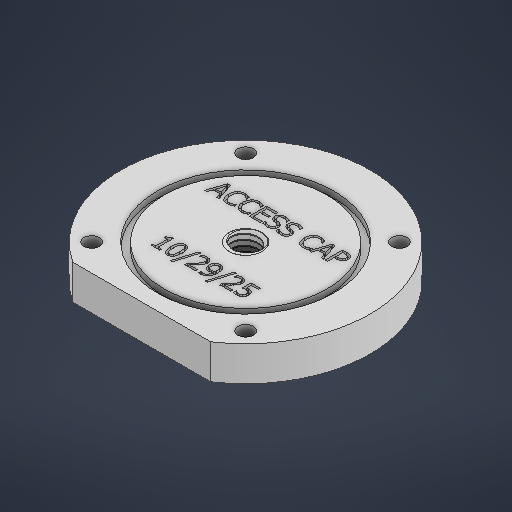
# Autodesk Inventor part: Access Cap
Saved by Autodesk Inventor 2026.2 (Build 302298000, 298)
## iProperties
Created: 2025-10-23
Part Number: Access Cap
Material: Generic
Document SubType Name: Modeling
Designer: mumin
Density: 1 g/cm^3
Appearance: Default
Author: mumin
Autodesk Inventor part; units mm, degrees
ref_plane "YZ Plane" through (0, 0, 0) normal (1, 0, 0) x (0, 1, 0)
ref_plane "XZ Plane" through (0, 0, 0) normal (0, 1, 0) x (-1, 0, 0)
ref_plane "XY Plane" through (0, 0, 0) normal (0, 0, 1) x (1, 0, 0)
sketch "Sketch1" plane through (0, 0, 0) normal (0, 1, 0) x (-1, 0, 0)
  circle A0 centre (0, 0) radius 36
  line L0 (19.8997, 30) -> (-19.8997, 30)
  dimension "d0" = 72
  dimension "d1" = 30
  constraints: 2 end point, 2 point on circle, 1 centre point, 1 coincident, 1 horizontal
  measures "d0" diameter of A0
  measures "d1" distance from line of point (0, 0) L0
extrude "Base" add sketch "Sketch1" along normal blind 10 contours A0 L0 picked at (-0.4083, 8.0069)
sketch "Sketch2" plane through (0, 0, 0) normal (0, -1, 0) x (1, 0, 0)
  circle A0 centre (0, 0) radius 31.4
  line L0 (22.2032, 22.2032) -> (0, 0)
  line L1 (-50.4, 0) -> (50.4, 0) projected
  dimension "d11" = 62.8
  dimension "d12" = 45
  constraints: 2 end point, 1 coincident, 3 other
  measures "d12" angle of L1 L0
hole "Mounting Holes" at (22.2032, 0, 22.2032) direction (0, 1, 0) diameter 4.5 end through all counterbore diameter 8 counterbore depth 4
pattern_circular "Circular Pattern1" count 4 over 360 about axis through (0, 0, 0) along (0, 1, 0) of "Mounting Holes"
sketch "Sketch3" plane through (0, 0, 0) normal (0, 0, 1) x (1, 0, 0)
  line L0 (36, 10) -> (-36, 10) projected
  line L1 (-25.5, 10) -> (-23.5, 10)
  line L2 (-23.5, 10) -> (-23.5, 8.2)
  line L3 (-23.5, 8.2) -> (-25.5, 8.2)
  line L4 (-25.5, 8.2) -> (-25.5, 10)
  line L5 (0, -2) -> (0, 12) projected
  point P0 (0, 0)
  point P1 (19.8997, 10)
  point P2 (-19.8997, 10)
  point P3 (0, 10)
  dimension "d16" = 2
  dimension "d17" = 1.8
  dimension "d18" = 23.5
  constraints: 8 end point, 2 parallel, 1 horizontal, 1 midpoint, 1 perpendicular, 1 point on line
  measures "d16" distance of L2.end L3.end
  measures "d17" distance of L1.end L2.end
  measures "d18" distance from line of point (0, 10) L2
revolve "Seal Groove" cut sketch "Sketch3" angle 360 about axis through (0, -10, 0) along (0, 1, 0)
sketch "Sketch4" plane through (0, 0, 0) normal (0, -1, 0) x (1, 0, 0)
  point P0 (0, 0)
  point P1 (0, 0)
  constraints: 1 coincident
hole "Wire Passthrough" at (0, 0, 0) direction (0, 1, 0) diameter 9.5 end through all
thread "Thread3" size "M10x1.5" class "6H" standard "ANSI Metric M Profile" length 10
sketch "Sketch14" plane through (0, 10, 0) normal (1, 0, 0) x (0, 0, 1)
  line L0 (4.75, 0) -> (4.75, 10)
  line L1 (4.75, 10) -> (3.6378, 10)
  line L2 (3.6378, 10) -> (3.6378, 0)
  line L3 (3.6378, 0) -> (4.75, 0)
  line L4 (0, -3.9629) -> (0, 12.3271) projected
  constraints: 8 end point
revolve "Revolution5" add sketch "Sketch14" angle 360 about axis through (0, 10, 0) along (0, -1, 0) separate body
sketch "Sketch13" plane through (0, 10, 4.75) normal (-1, 0, 0) x (0, -1, 0)
  line L0 (-0.8751, -0.076) -> (-0.7501, -0.076) construction
  line L1 (0.1249, -1.0365) -> (-0.0001, -1.2766) construction
  line L2 (-1.5001, -1.2766) -> (-1.6251, -1.0365) construction
  line L3 (-0.6251, -0.076) -> (-0.7501, 0.1641) construction
  line L4 (-0.7501, 0.1641) -> (-0.8751, -0.076) construction
  line L5 (-1.5001, -1.2766) -> (-1.3751, -1.0365) construction
  line L6 (-0.6251, -0.076) -> (-0.1251, -1.0365)
  line L7 (-1.6251, -1.0365) -> (-1.3751, -1.0365) construction
  arc A0 (-1.6251, -1.0365) -> (-1.5001, -1.1124) centre (-1.5001, -0.9714) ccw construction
  line L8 (0.1249, -1.0365) -> (-0.1251, -1.0365) construction
  line L9 (-1.5001, -1.2766) -> (-1.5001, -1.0365) construction
  line L10 (-0.0001, -1.2766) -> (-0.0001, -1.0365) construction
  line L11 (-0.7501, 0.1641) -> (-0.7501, -0.0002) construction
  line L12 (-1.5001, -1.1124) -> (-0.0001, -1.1124)
  arc A1 (-1.5001, -1.1124) -> (-1.3751, -1.0365) centre (-1.5001, -0.9714) ccw
  line L13 (-0.1251, -1.0365) -> (-0.0001, -1.2766) construction
  line L14 (-1.3751, -1.0365) -> (-0.8751, -0.076)
  line L15 (-0.0001, -0.0002) -> (-0.0001, 0.0177)
  line L16 (-0.0001, 0.0177) -> (-0.0001, -0.0002)
  line L17 (-0.0001, -0.0002) -> (0.0334, -0.0002)
  arc A2 (-0.1251, -1.0365) -> (-0.0001, -1.1124) centre (-0.0001, -0.9714) ccw
  arc A3 (-0.0001, -1.1124) -> (0.1249, -1.0365) centre (-0.0001, -0.9714) ccw construction
  arc A4 (-0.7501, -0.0002) -> (-0.8751, -0.076) centre (-0.7501, -0.1411) ccw
  arc A5 (-0.6251, -0.076) -> (-0.7501, -0.0002) centre (-0.7501, -0.1411) ccw
  line L18 (-0.7501, -0.0002) -> (-0.7501, -0.076) construction
  line L19 (-0.7501, -0.076) -> (-0.6251, -0.076) construction
  dimension "d87" = 55
  dimension "d88" = 0.2401
  dimension "d89" = 0.2401
  dimension "Sketch13_ThreadOffset" = 0
  dimension "Sketch13_MajorRadius" = 1.1122
  dimension "d92" = 1.5
  dimension "Sketch13_MinorRadius" = 0
  constraints: 40 end point, 12 point on circle, 10 parallel, 8 tangent, 6 centre point, 6 collinear, 2 midpoint, 2 point on line, 1 horizontal, 1 perpendicular, 3 other
  measures "d87" angle of L6 L14
  measures "d88" distance of L3.end L0.end
  measures "d89" distance of L1.end L10.end
  measures "Sketch13_ThreadOffset" distance between parallel lines of L15 L10
  measures "Sketch13_MajorRadius" distance from line of L12 L15.start
  measures "d92" distance from line of L1.end L9
  measures "Sketch13_MinorRadius" distance edge to line of A5 L17
coil "Coil4" sketch "Sketch13" operation cut axis through (0, 10, 0) along (0, -1, 0) pitch 1.5015 turns 8.658009 hand right bodies 2
sketch "Sketch15" plane through (0, 10, 0) normal (0, 1, 0) x (1, 0, 0)
  line L0 (-18.801, 12.0638) -> (19.2906, 12.0638) construction
  line L1 (19.2906, 12.0638) -> (19.2906, -2.3437) construction
  line L2 (19.2906, -2.3437) -> (-18.801, -2.3437) construction
  line L3 (-18.801, -2.3437) -> (-18.801, 12.0638) construction
  line L4 (-18.8334, 6.9746) -> (-17.1479, 11.9746)
  line L5 (-17.1479, 11.9746) -> (-16.3294, 11.9746)
  line L6 (-16.3294, 11.9746) -> (-14.6438, 6.9746)
  line L7 (-14.6438, 6.9746) -> (-15.3448, 6.9746)
  line L8 (-15.3448, 6.9746) -> (-15.7986, 8.3725)
  line L9 (-15.7986, 8.3725) -> (-17.707, 8.3725)
  line L10 (-17.707, 8.3725) -> (-18.1608, 6.9746)
  line L11 (-18.1608, 6.9746) -> (-18.8334, 6.9746)
  line L12 (-15.9809, 8.9398) -> (-16.7548, 11.2939)
  line L13 (-16.7548, 11.2939) -> (-17.5247, 8.9398)
  line L14 (-17.5247, 8.9398) -> (-15.9809, 8.9398)
  spline S0 degree 2 poles (-12.2167, 6.8855) (-12.703, 6.8855) (-13.5255, 7.2137) (-13.8253, 7.5419) knots 0 0 0 1 2 2 2
  spline S1 degree 2 poles (-13.8253, 7.5419) (-14.1252, 7.866) (-14.4534, 8.8385) (-14.4534, 9.4706) knots 0 0 0 1 2 2 2
  spline S2 degree 2 poles (-14.4534, 9.4706) (-14.4534, 10.0986) (-14.1333, 11.0305) (-13.8294, 11.3749) knots 0 0 0 1 2 2 2
  spline S3 degree 2 poles (-13.8294, 11.3749) (-13.5295, 11.7112) (-12.7111, 12.0638) (-12.2046, 12.0638) knots 0 0 0 1 2 2 2
  spline S4 degree 2 poles (-12.2046, 12.0638) (-11.9534, 12.0638) (-11.5117, 11.9908) (-11.3253, 11.9341) knots 0 0 0 1 2 2 2
  spline S5 degree 2 poles (-11.3253, 11.9341) (-11.1633, 11.8814) (-10.8269, 11.7315) (-10.6608, 11.6424) knots 0 0 0 1 2 2 2
  line L15 (-10.6608, 11.6424) -> (-10.6608, 10.8401)
  line L16 (-10.6608, 10.8401) -> (-10.7135, 10.8401)
  spline S6 degree 2 poles (-10.7135, 10.8401) (-10.8026, 10.9211) (-11.0782, 11.148) (-11.2767, 11.2574) knots 0 0 0 1 2 2 2
  spline S7 degree 2 poles (-11.2767, 11.2574) (-11.4671, 11.3628) (-11.9169, 11.4965) (-12.2086, 11.4965) knots 0 0 0 1 2 2 2
  spline S8 degree 2 poles (-12.2086, 11.4965) (-12.5287, 11.4965) (-13.1, 11.2331) (-13.3148, 10.9819) knots 0 0 0 1 2 2 2
  spline S9 degree 2 poles (-13.3148, 10.9819) (-13.5255, 10.7266) (-13.7605, 9.9527) (-13.7605, 9.4706) knots 0 0 0 1 2 2 2
  spline S10 degree 2 poles (-13.7605, 9.4706) (-13.7605, 8.956) (-13.5133, 8.2145) (-13.2986, 7.9592) knots 0 0 0 1 2 2 2
  spline S11 degree 2 poles (-13.2986, 7.9592) (-13.0879, 7.7121) (-12.5247, 7.4608) (-12.2086, 7.4608) knots 0 0 0 1 2 2 2
  spline S12 degree 2 poles (-12.2086, 7.4608) (-11.9209, 7.4608) (-11.4307, 7.6027) (-11.2402, 7.708) knots 0 0 0 1 2 2 2
  spline S13 degree 2 poles (-11.2402, 7.708) (-11.0579, 7.8133) (-10.7864, 8.0321) (-10.7094, 8.1091) knots 0 0 0 1 2 2 2
  line L17 (-10.7094, 8.1091) -> (-10.6608, 8.1091)
  line L18 (-10.6608, 8.1091) -> (-10.6608, 7.315)
  spline S14 degree 2 poles (-10.6608, 7.315) (-10.8269, 7.238) (-11.1187, 7.0962) (-11.3253, 7.0313) knots 0 0 0 1 2 2 2
  spline S15 degree 2 poles (-11.3253, 7.0313) (-11.5441, 6.9584) (-11.9169, 6.8855) (-12.2167, 6.8855) knots 0 0 0 1 2 2 2
  spline S16 degree 2 poles (-8.0879, 6.8855) (-8.5741, 6.8855) (-9.3966, 7.2137) (-9.6965, 7.5419) knots 0 0 0 1 2 2 2
  spline S17 degree 2 poles (-9.6965, 7.5419) (-9.9963, 7.866) (-10.3245, 8.8385) (-10.3245, 9.4706) knots 0 0 0 1 2 2 2
  spline S18 degree 2 poles (-10.3245, 9.4706) (-10.3245, 10.0986) (-10.0044, 11.0305) (-9.7005, 11.3749) knots 0 0 0 1 2 2 2
  spline S19 degree 2 poles (-9.7005, 11.3749) (-9.4007, 11.7112) (-8.5822, 12.0638) (-8.0757, 12.0638) knots 0 0 0 1 2 2 2
  spline S20 degree 2 poles (-8.0757, 12.0638) (-7.8245, 12.0638) (-7.3829, 11.9908) (-7.1965, 11.9341) knots 0 0 0 1 2 2 2
  spline S21 degree 2 poles (-7.1965, 11.9341) (-7.0344, 11.8814) (-6.6981, 11.7315) (-6.532, 11.6424) knots 0 0 0 1 2 2 2
  line L19 (-6.532, 11.6424) -> (-6.532, 10.8401)
  line L20 (-6.532, 10.8401) -> (-6.5846, 10.8401)
  spline S22 degree 2 poles (-6.5846, 10.8401) (-6.6738, 10.9211) (-6.9493, 11.148) (-7.1479, 11.2574) knots 0 0 0 1 2 2 2
  spline S23 degree 2 poles (-7.1479, 11.2574) (-7.3383, 11.3628) (-7.788, 11.4965) (-8.0798, 11.4965) knots 0 0 0 1 2 2 2
  spline S24 degree 2 poles (-8.0798, 11.4965) (-8.3999, 11.4965) (-8.9712, 11.2331) (-9.1859, 10.9819) knots 0 0 0 1 2 2 2
  spline S25 degree 2 poles (-9.1859, 10.9819) (-9.3966, 10.7266) (-9.6316, 9.9527) (-9.6316, 9.4706) knots 0 0 0 1 2 2 2
  spline S26 degree 2 poles (-9.6316, 9.4706) (-9.6316, 8.956) (-9.3845, 8.2145) (-9.1697, 7.9592) knots 0 0 0 1 2 2 2
  spline S27 degree 2 poles (-9.1697, 7.9592) (-8.959, 7.7121) (-8.3958, 7.4608) (-8.0798, 7.4608) knots 0 0 0 1 2 2 2
  spline S28 degree 2 poles (-8.0798, 7.4608) (-7.7921, 7.4608) (-7.3018, 7.6027) (-7.1114, 7.708) knots 0 0 0 1 2 2 2
  spline S29 degree 2 poles (-7.1114, 7.708) (-6.9291, 7.8133) (-6.6576, 8.0321) (-6.5806, 8.1091) knots 0 0 0 1 2 2 2
  line L21 (-6.5806, 8.1091) -> (-6.532, 8.1091)
  line L22 (-6.532, 8.1091) -> (-6.532, 7.315)
  spline S30 degree 2 poles (-6.532, 7.315) (-6.6981, 7.238) (-6.9898, 7.0962) (-7.1965, 7.0313) knots 0 0 0 1 2 2 2
  spline S31 degree 2 poles (-7.1965, 7.0313) (-7.4153, 6.9584) (-7.788, 6.8855) (-8.0879, 6.8855) knots 0 0 0 1 2 2 2
  line L23 (-5.912, 6.9746) -> (-5.912, 11.9746)
  line L24 (-5.912, 11.9746) -> (-2.784, 11.9746)
  line L25 (-2.784, 11.9746) -> (-2.784, 11.383)
  line L26 (-2.784, 11.383) -> (-5.2475, 11.383)
  line L27 (-5.2475, 11.383) -> (-5.2475, 10.0135)
  line L28 (-5.2475, 10.0135) -> (-2.9501, 10.0135)
  line L29 (-2.9501, 10.0135) -> (-2.9501, 9.4219)
  line L30 (-2.9501, 9.4219) -> (-5.2475, 9.4219)
  line L31 (-5.2475, 9.4219) -> (-5.2475, 7.5662)
  line L32 (-5.2475, 7.5662) -> (-2.784, 7.5662)
  line L33 (-2.784, 7.5662) -> (-2.784, 6.9746)
  line L34 (-2.784, 6.9746) -> (-5.912, 6.9746)
  spline S32 degree 2 poles (-0.6608, 6.8855) (-1.2038, 6.8855) (-1.9655, 7.1124) (-2.3018, 7.2745) knots 0 0 0 1 2 2 2
  line L35 (-2.3018, 7.2745) -> (-2.3018, 8.1091)
  line L36 (-2.3018, 8.1091) -> (-2.2532, 8.1091)
  spline S33 degree 2 poles (-2.2532, 8.1091) (-1.925, 7.8012) (-1.0944, 7.4608) (-0.7094, 7.4608) knots 0 0 0 1 2 2 2
  spline S34 degree 2 poles (-0.7094, 7.4608) (-0.1584, 7.4608) (0.4048, 7.9187) (0.4048, 8.2955) knots 0 0 0 1 2 2 2
  spline S35 degree 2 poles (0.4048, 8.2955) (0.4048, 8.5954) (0.109, 8.9681) (-0.2111, 9.0613) knots 0 0 0 1 2 2 2
  spline S36 degree 2 poles (-0.2111, 9.0613) (-0.442, 9.1262) (-0.8269, 9.2153) (-1.1146, 9.2882) knots 0 0 0 1 2 2 2
  spline S37 degree 2 poles (-1.1146, 9.2882) (-1.3739, 9.3571) (-1.7832, 9.5638) (-1.9412, 9.7299) knots 0 0 0 1 2 2 2
  spline S38 degree 2 poles (-1.9412, 9.7299) (-2.0952, 9.896) (-2.2654, 10.3417) (-2.2654, 10.6334) knots 0 0 0 1 2 2 2
  spline S39 degree 2 poles (-2.2654, 10.6334) (-2.2654, 11.2412) (-1.3172, 12.0638) (-0.5838, 12.0638) knots 0 0 0 1 2 2 2
  spline S40 degree 2 poles (-0.5838, 12.0638) (-0.1624, 12.0638) (0.5831, 11.8976) (0.9032, 11.7396) knots 0 0 0 1 2 2 2
  line L37 (0.9032, 11.7396) -> (0.9032, 10.9454)
  line L38 (0.9032, 10.9454) -> (0.8546, 10.9454)
  spline S41 degree 2 poles (0.8546, 10.9454) (0.6155, 11.1642) (-0.13, 11.4884) (-0.5393, 11.4884) knots 0 0 0 1 2 2 2
  spline S42 degree 2 poles (-0.5393, 11.4884) (-1.0012, 11.4884) (-1.5725, 11.0548) (-1.5725, 10.7023) knots 0 0 0 1 2 2 2
  spline S43 degree 2 poles (-1.5725, 10.7023) (-1.5725, 10.3863) (-1.2362, 10.0095) (-0.9201, 9.9244) knots 0 0 0 1 2 2 2
  spline S44 degree 2 poles (-0.9201, 9.9244) (-0.7094, 9.8676) (-0.0976, 9.7218) (0.105, 9.661) knots 0 0 0 1 2 2 2
  spline S45 degree 2 poles (0.105, 9.661) (0.6196, 9.503) (1.0977, 8.8668) (1.0977, 8.4009) knots 0 0 0 1 2 2 2
  spline S46 degree 2 poles (1.0977, 8.4009) (1.0977, 8.1051) (0.8586, 7.5378) (0.6439, 7.3393) knots 0 0 0 1 2 2 2
  spline S47 degree 2 poles (0.6439, 7.3393) (0.4048, 7.1205) (-0.203, 6.8855) (-0.6608, 6.8855) knots 0 0 0 1 2 2 2
  spline S48 degree 2 poles (3.1682, 6.8855) (2.6252, 6.8855) (1.8635, 7.1124) (1.5272, 7.2745) knots 0 0 0 1 2 2 2
  line L39 (1.5272, 7.2745) -> (1.5272, 8.1091)
  line L40 (1.5272, 8.1091) -> (1.5758, 8.1091)
  spline S49 degree 2 poles (1.5758, 8.1091) (1.904, 7.8012) (2.7346, 7.4608) (3.1196, 7.4608) knots 0 0 0 1 2 2 2
  spline S50 degree 2 poles (3.1196, 7.4608) (3.6706, 7.4608) (4.2338, 7.9187) (4.2338, 8.2955) knots 0 0 0 1 2 2 2
  spline S51 degree 2 poles (4.2338, 8.2955) (4.2338, 8.5954) (3.938, 8.9681) (3.6179, 9.0613) knots 0 0 0 1 2 2 2
  spline S52 degree 2 poles (3.6179, 9.0613) (3.387, 9.1262) (3.0021, 9.2153) (2.7144, 9.2882) knots 0 0 0 1 2 2 2
  spline S53 degree 2 poles (2.7144, 9.2882) (2.4551, 9.3571) (2.0458, 9.5638) (1.8878, 9.7299) knots 0 0 0 1 2 2 2
  spline S54 degree 2 poles (1.8878, 9.7299) (1.7338, 9.896) (1.5637, 10.3417) (1.5637, 10.6334) knots 0 0 0 1 2 2 2
  spline S55 degree 2 poles (1.5637, 10.6334) (1.5637, 11.2412) (2.5118, 12.0638) (3.2452, 12.0638) knots 0 0 0 1 2 2 2
  spline S56 degree 2 poles (3.2452, 12.0638) (3.6666, 12.0638) (4.4121, 11.8976) (4.7322, 11.7396) knots 0 0 0 1 2 2 2
  line L41 (4.7322, 11.7396) -> (4.7322, 10.9454)
  line L42 (4.7322, 10.9454) -> (4.6836, 10.9454)
  spline S57 degree 2 poles (4.6836, 10.9454) (4.4445, 11.1642) (3.699, 11.4884) (3.2897, 11.4884) knots 0 0 0 1 2 2 2
  spline S58 degree 2 poles (3.2897, 11.4884) (2.8278, 11.4884) (2.2565, 11.0548) (2.2565, 10.7023) knots 0 0 0 1 2 2 2
  spline S59 degree 2 poles (2.2565, 10.7023) (2.2565, 10.3863) (2.5928, 10.0095) (2.9089, 9.9244) knots 0 0 0 1 2 2 2
  spline S60 degree 2 poles (2.9089, 9.9244) (3.1196, 9.8676) (3.7314, 9.7218) (3.934, 9.661) knots 0 0 0 1 2 2 2
  spline S61 degree 2 poles (3.934, 9.661) (4.4486, 9.503) (4.9267, 8.8668) (4.9267, 8.4009) knots 0 0 0 1 2 2 2
  spline S62 degree 2 poles (4.9267, 8.4009) (4.9267, 8.1051) (4.6876, 7.5378) (4.4729, 7.3393) knots 0 0 0 1 2 2 2
  spline S63 degree 2 poles (4.4729, 7.3393) (4.2338, 7.1205) (3.6261, 6.8855) (3.1682, 6.8855) knots 0 0 0 1 2 2 2
  spline S64 degree 2 poles (9.7038, 6.8855) (9.2176, 6.8855) (8.3951, 7.2137) (8.0953, 7.5419) knots 0 0 0 1 2 2 2
  spline S65 degree 2 poles (8.0953, 7.5419) (7.7954, 7.866) (7.4672, 8.8385) (7.4672, 9.4706) knots 0 0 0 1 2 2 2
  spline S66 degree 2 poles (7.4672, 9.4706) (7.4672, 10.0986) (7.7873, 11.0305) (8.0912, 11.3749) knots 0 0 0 1 2 2 2
  spline S67 degree 2 poles (8.0912, 11.3749) (8.391, 11.7112) (9.2095, 12.0638) (9.716, 12.0638) knots 0 0 0 1 2 2 2
  spline S68 degree 2 poles (9.716, 12.0638) (9.9672, 12.0638) (10.4089, 11.9908) (10.5953, 11.9341) knots 0 0 0 1 2 2 2
  spline S69 degree 2 poles (10.5953, 11.9341) (10.7573, 11.8814) (11.0936, 11.7315) (11.2598, 11.6424) knots 0 0 0 1 2 2 2
  line L43 (11.2598, 11.6424) -> (11.2598, 10.8401)
  line L44 (11.2598, 10.8401) -> (11.2071, 10.8401)
  spline S70 degree 2 poles (11.2071, 10.8401) (11.1179, 10.9211) (10.8424, 11.148) (10.6439, 11.2574) knots 0 0 0 1 2 2 2
  spline S71 degree 2 poles (10.6439, 11.2574) (10.4534, 11.3628) (10.0037, 11.4965) (9.712, 11.4965) knots 0 0 0 1 2 2 2
  spline S72 degree 2 poles (9.712, 11.4965) (9.3919, 11.4965) (8.8205, 11.2331) (8.6058, 10.9819) knots 0 0 0 1 2 2 2
  spline S73 degree 2 poles (8.6058, 10.9819) (8.3951, 10.7266) (8.1601, 9.9527) (8.1601, 9.4706) knots 0 0 0 1 2 2 2
  spline S74 degree 2 poles (8.1601, 9.4706) (8.1601, 8.956) (8.4073, 8.2145) (8.622, 7.9592) knots 0 0 0 1 2 2 2
  spline S75 degree 2 poles (8.622, 7.9592) (8.8327, 7.7121) (9.3959, 7.4608) (9.712, 7.4608) knots 0 0 0 1 2 2 2
  spline S76 degree 2 poles (9.712, 7.4608) (9.9996, 7.4608) (10.4899, 7.6027) (10.6803, 7.708) knots 0 0 0 1 2 2 2
  spline S77 degree 2 poles (10.6803, 7.708) (10.8627, 7.8133) (11.1342, 8.0321) (11.2111, 8.1091) knots 0 0 0 1 2 2 2
  line L45 (11.2111, 8.1091) -> (11.2598, 8.1091)
  line L46 (11.2598, 8.1091) -> (11.2598, 7.315)
  spline S78 degree 2 poles (11.2598, 7.315) (11.0936, 7.238) (10.8019, 7.0962) (10.5953, 7.0313) knots 0 0 0 1 2 2 2
  spline S79 degree 2 poles (10.5953, 7.0313) (10.3765, 6.9584) (10.0037, 6.8855) (9.7038, 6.8855) knots 0 0 0 1 2 2 2
  line L47 (11.3408, 6.9746) -> (13.0264, 11.9746)
  line L48 (13.0264, 11.9746) -> (13.8449, 11.9746)
  line L49 (13.8449, 11.9746) -> (15.5304, 6.9746)
  line L50 (15.5304, 6.9746) -> (14.8295, 6.9746)
  line L51 (14.8295, 6.9746) -> (14.3756, 8.3725)
  line L52 (14.3756, 8.3725) -> (12.4672, 8.3725)
  line L53 (12.4672, 8.3725) -> (12.0134, 6.9746)
  line L54 (12.0134, 6.9746) -> (11.3408, 6.9746)
  line L55 (14.1933, 8.9398) -> (13.4194, 11.2939)
  line L56 (13.4194, 11.2939) -> (12.6496, 8.9398)
  line L57 (12.6496, 8.9398) -> (14.1933, 8.9398)
  spline S80 degree 2 poles (19.165, 10.4673) (19.165, 10.1432) (18.934, 9.5597) (18.7273, 9.3571) knots 0 0 0 1 2 2 2
  spline S81 degree 2 poles (18.7273, 9.3571) (18.468, 9.1018) (17.7671, 8.8385) (17.2322, 8.8385) knots 0 0 0 1 2 2 2
  line L58 (17.2322, 8.8385) -> (16.669, 8.8385)
  line L59 (16.669, 8.8385) -> (16.669, 6.9746)
  line L60 (16.669, 6.9746) -> (16.0045, 6.9746)
  line L61 (16.0045, 6.9746) -> (16.0045, 11.9746)
  line L62 (16.0045, 11.9746) -> (17.2606, 11.9746)
  spline S82 degree 2 poles (17.2606, 11.9746) (17.7063, 11.9746) (18.3303, 11.8287) (18.5693, 11.6626) knots 0 0 0 1 2 2 2
  spline S83 degree 2 poles (18.5693, 11.6626) (18.8489, 11.4722) (19.165, 10.8847) (19.165, 10.4673) knots 0 0 0 1 2 2 2
  spline S84 degree 2 poles (18.4721, 10.4471) (18.4721, 10.7064) (18.2938, 11.0873) (18.1115, 11.2088) knots 0 0 0 1 2 2 2
  spline S85 degree 2 poles (18.1115, 11.2088) (17.9534, 11.3142) (17.532, 11.3992) (17.2201, 11.3992) knots 0 0 0 1 2 2 2
  line L63 (17.2201, 11.3992) -> (16.669, 11.3992)
  line L64 (16.669, 11.3992) -> (16.669, 9.4057)
  line L65 (16.669, 9.4057) -> (17.1228, 9.4057)
  spline S86 degree 2 poles (17.1228, 9.4057) (17.528, 9.4057) (18.0264, 9.5354) (18.1885, 9.7056) knots 0 0 0 1 2 2 2
  spline S87 degree 2 poles (18.1885, 9.7056) (18.3384, 9.8555) (18.4721, 10.208) (18.4721, 10.4471) knots 0 0 0 1 2 2 2
  line L66 (-10.444, -14.4295) -> (-12.8833, -14.4295)
  line L67 (-12.8833, -14.4295) -> (-12.8833, -13.919)
  line L68 (-12.8833, -13.919) -> (-11.9756, -13.919)
  line L69 (-11.9756, -13.919) -> (-11.9756, -10.5681)
  line L70 (-11.9756, -10.5681) -> (-12.8833, -10.5681)
  line L71 (-12.8833, -10.5681) -> (-12.8833, -10.1103)
  spline S88 degree 2 poles (-12.8833, -10.1103) (-12.3687, -10.1103) (-11.8825, -9.8185) (-11.85, -9.4133) knots 0 0 0 1 2 2 2
  line L72 (-11.85, -9.4133) -> (-11.3314, -9.4133)
  line L73 (-11.3314, -9.4133) -> (-11.3314, -13.919)
  line L74 (-11.3314, -13.919) -> (-10.444, -13.919)
  line L75 (-10.444, -13.919) -> (-10.444, -14.4295)
  spline S89 degree 2 poles (-6.4124, -11.9295) (-6.4124, -13.2748) (-7.1945, -14.5349) (-8.0089, -14.5349) knots 0 0 0 1 2 2 2
  spline S90 degree 2 poles (-8.0089, -14.5349) (-8.8355, -14.5349) (-9.6094, -13.2505) (-9.6094, -11.9336) knots 0 0 0 1 2 2 2
  spline S91 degree 2 poles (-9.6094, -11.9336) (-9.6094, -10.5803) (-8.8274, -9.3282) (-8.0089, -9.3282) knots 0 0 0 1 2 2 2
  spline S92 degree 2 poles (-8.0089, -9.3282) (-7.1863, -9.3282) (-6.4124, -10.6248) (-6.4124, -11.9295) knots 0 0 0 1 2 2 2
  spline S93 degree 2 poles (-7.2714, -13.453) (-7.1742, -13.2059) (-7.0932, -12.4441) (-7.0932, -11.9295) knots 0 0 0 1 2 2 2
  spline S94 degree 2 poles (-7.0932, -11.9295) (-7.0932, -11.415) (-7.1742, -10.6573) (-7.2755, -10.402) knots 0 0 0 1 2 2 2
  spline S95 degree 2 poles (-7.2755, -10.402) (-7.3768, -10.1467) (-7.7293, -9.8834) (-8.0089, -9.8834) knots 0 0 0 1 2 2 2
  spline S96 degree 2 poles (-8.0089, -9.8834) (-8.2885, -9.8834) (-8.6491, -10.1467) (-8.7544, -10.4101) knots 0 0 0 1 2 2 2
  spline S97 degree 2 poles (-8.7544, -10.4101) (-8.8557, -10.6654) (-8.9286, -11.4433) (-8.9286, -11.9336) knots 0 0 0 1 2 2 2
  spline S98 degree 2 poles (-8.9286, -11.9336) (-8.9286, -12.4603) (-8.8638, -13.1654) (-8.7585, -13.4409) knots 0 0 0 1 2 2 2
  spline S99 degree 2 poles (-8.7585, -13.4409) (-8.6612, -13.7002) (-8.3006, -13.9798) (-8.0089, -13.9798) knots 0 0 0 1 2 2 2
  spline S100 degree 2 poles (-8.0089, -13.9798) (-7.7333, -13.9798) (-7.3727, -13.7164) (-7.2714, -13.453) knots 0 0 0 1 2 2 2
  line L76 (-3.6936, -9.2067) -> (-5.6507, -15.5154)
  line L77 (-5.6507, -15.5154) -> (-6.218, -15.5154)
  line L78 (-6.218, -15.5154) -> (-4.269, -9.2067)
  line L79 (-4.269, -9.2067) -> (-3.6936, -9.2067)
  line L80 (-0.0591, -14.4295) -> (-3.1426, -14.4295)
  line L81 (-3.1426, -14.4295) -> (-3.1426, -13.7205)
  spline S101 degree 2 poles (-3.1426, -13.7205) (-2.8103, -13.4085) (-2.2188, -12.8291) (-1.9351, -12.5171) knots 0 0 0 1 2 2 2
  spline S102 degree 2 poles (-1.9351, -12.5171) (-1.3638, -11.889) (-0.9465, -11.1354) (-0.9465, -10.7342) knots 0 0 0 1 2 2 2
  spline S103 degree 2 poles (-0.9465, -10.7342) (-0.9465, -10.5235) (-1.0761, -10.2075) (-1.1936, -10.1062) knots 0 0 0 1 2 2 2
  spline S104 degree 2 poles (-1.1936, -10.1062) (-1.3111, -10.0049) (-1.6191, -9.9036) (-1.8055, -9.9036) knots 0 0 0 1 2 2 2
  spline S105 degree 2 poles (-1.8055, -9.9036) (-1.9838, -9.9036) (-2.3484, -9.9928) (-2.5145, -10.0616) knots 0 0 0 1 2 2 2
  spline S106 degree 2 poles (-2.5145, -10.0616) (-2.6564, -10.1184) (-2.9197, -10.2804) (-3.0008, -10.3372) knots 0 0 0 1 2 2 2
  line L82 (-3.0008, -10.3372) -> (-3.0372, -10.3372)
  line L83 (-3.0372, -10.3372) -> (-3.0372, -9.624)
  spline S107 degree 2 poles (-3.0372, -9.624) (-2.8306, -9.5227) (-2.0891, -9.3242) (-1.7568, -9.3242) knots 0 0 0 1 2 2 2
  spline S108 degree 2 poles (-1.7568, -9.3242) (-1.0559, -9.3242) (-0.2658, -10.0657) (-0.2658, -10.6978) knots 0 0 0 1 2 2 2
  spline S109 degree 2 poles (-0.2658, -10.6978) (-0.2658, -10.9936) (-0.4035, -11.4879) (-0.5251, -11.6986) knots 0 0 0 1 2 2 2
  spline S110 degree 2 poles (-0.5251, -11.6986) (-0.6466, -11.9174) (-0.9992, -12.3469) (-1.1936, -12.5535) knots 0 0 0 1 2 2 2
  spline S111 degree 2 poles (-1.1936, -12.5535) (-1.5097, -12.8979) (-2.2836, -13.6354) (-2.5145, -13.8501) knots 0 0 0 1 2 2 2
  line L84 (-2.5145, -13.8501) -> (-0.0591, -13.8501)
  line L85 (-0.0591, -13.8501) -> (-0.0591, -14.4295)
  spline S112 degree 2 poles (0.4717, -11.0543) (0.4717, -10.6694) (0.7229, -10.0292) (0.9417, -9.7983) knots 0 0 0 1 2 2 2
  spline S113 degree 2 poles (0.9417, -9.7983) (1.1483, -9.5754) (1.7521, -9.3282) (2.06, -9.3282) knots 0 0 0 1 2 2 2
  spline S114 degree 2 poles (2.06, -9.3282) (2.4044, -9.3282) (2.9636, -9.5592) (3.1702, -9.778) knots 0 0 0 1 2 2 2
  spline S115 degree 2 poles (3.1702, -9.778) (3.4295, -10.0535) (3.7132, -10.9449) (3.7132, -11.6297) knots 0 0 0 1 2 2 2
  spline S116 degree 2 poles (3.7132, -11.6297) (3.7132, -12.2496) (3.4336, -13.3599) (3.1621, -13.7286) knots 0 0 0 1 2 2 2
  spline S117 degree 2 poles (3.1621, -13.7286) (2.8744, -14.1176) (2.0641, -14.5268) (1.4725, -14.5268) knots 0 0 0 1 2 2 2
  spline S118 degree 2 poles (1.4725, -14.5268) (1.3388, -14.5268) (1.0349, -14.4984) (0.9052, -14.4579) knots 0 0 0 1 2 2 2
  line L86 (0.9052, -14.4579) -> (0.9052, -13.8137)
  line L87 (0.9052, -13.8137) -> (0.9376, -13.8137)
  spline S119 degree 2 poles (0.9376, -13.8137) (1.0227, -13.8623) (1.3793, -13.9474) (1.5616, -13.9474) knots 0 0 0 1 2 2 2
  spline S120 degree 2 poles (1.5616, -13.9474) (2.218, -13.9474) (2.9676, -13.0803) (3.0203, -12.278) knots 0 0 0 1 2 2 2
  spline S121 degree 2 poles (3.0203, -12.278) (2.7529, -12.4603) (2.2667, -12.6265) (1.979, -12.6265) knots 0 0 0 1 2 2 2
  spline S122 degree 2 poles (1.979, -12.6265) (1.7034, -12.6265) (1.2456, -12.5049) (1.0146, -12.3307) knots 0 0 0 1 2 2 2
  spline S123 degree 2 poles (1.0146, -12.3307) (0.7472, -12.124) (0.4717, -11.496) (0.4717, -11.0543) knots 0 0 0 1 2 2 2
  spline S124 degree 2 poles (3.0365, -11.4798) (3.0365, -10.9733) (2.8501, -10.3331) (2.684, -10.1589) knots 0 0 0 1 2 2 2
  spline S125 degree 2 poles (2.684, -10.1589) (2.5381, -9.9968) (2.2342, -9.8752) (2.056, -9.8752) knots 0 0 0 1 2 2 2
  spline S126 degree 2 poles (2.056, -9.8752) (1.6427, -9.8752) (1.1524, -10.4668) (1.1524, -11.026) knots 0 0 0 1 2 2 2
  spline S127 degree 2 poles (1.1524, -11.026) (1.1524, -11.342) (1.3145, -11.7513) (1.4927, -11.8971) knots 0 0 0 1 2 2 2
  spline S128 degree 2 poles (1.4927, -11.8971) (1.6224, -12.0025) (1.9425, -12.0714) (2.1289, -12.0714) knots 0 0 0 1 2 2 2
  spline S129 degree 2 poles (2.1289, -12.0714) (2.3436, -12.0714) (2.838, -11.9214) (3.0244, -11.7958) knots 0 0 0 1 2 2 2
  spline S130 degree 2 poles (3.0244, -11.7958) (3.0284, -11.7472) (3.0365, -11.5811) (3.0365, -11.4798) knots 0 0 0 1 2 2 2
  line L88 (6.4401, -9.2067) -> (4.483, -15.5154)
  line L89 (4.483, -15.5154) -> (3.9158, -15.5154)
  line L90 (3.9158, -15.5154) -> (5.8647, -9.2067)
  line L91 (5.8647, -9.2067) -> (6.4401, -9.2067)
  line L92 (10.0746, -14.4295) -> (6.9911, -14.4295)
  line L93 (6.9911, -14.4295) -> (6.9911, -13.7205)
  spline S131 degree 2 poles (6.9911, -13.7205) (7.3234, -13.4085) (7.9149, -12.8291) (8.1986, -12.5171) knots 0 0 0 1 2 2 2
  spline S132 degree 2 poles (8.1986, -12.5171) (8.7699, -11.889) (9.1872, -11.1354) (9.1872, -10.7342) knots 0 0 0 1 2 2 2
  spline S133 degree 2 poles (9.1872, -10.7342) (9.1872, -10.5235) (9.0576, -10.2075) (8.9401, -10.1062) knots 0 0 0 1 2 2 2
  spline S134 degree 2 poles (8.9401, -10.1062) (8.8226, -10.0049) (8.5146, -9.9036) (8.3282, -9.9036) knots 0 0 0 1 2 2 2
  spline S135 degree 2 poles (8.3282, -9.9036) (8.15, -9.9036) (7.7853, -9.9928) (7.6192, -10.0616) knots 0 0 0 1 2 2 2
  spline S136 degree 2 poles (7.6192, -10.0616) (7.4773, -10.1184) (7.214, -10.2804) (7.1329, -10.3372) knots 0 0 0 1 2 2 2
  line L94 (7.1329, -10.3372) -> (7.0965, -10.3372)
  line L95 (7.0965, -10.3372) -> (7.0965, -9.624)
  spline S137 degree 2 poles (7.0965, -9.624) (7.3031, -9.5227) (8.0446, -9.3242) (8.3769, -9.3242) knots 0 0 0 1 2 2 2
  spline S138 degree 2 poles (8.3769, -9.3242) (9.0778, -9.3242) (9.8679, -10.0657) (9.8679, -10.6978) knots 0 0 0 1 2 2 2
  spline S139 degree 2 poles (9.8679, -10.6978) (9.8679, -10.9936) (9.7302, -11.4879) (9.6086, -11.6986) knots 0 0 0 1 2 2 2
  spline S140 degree 2 poles (9.6086, -11.6986) (9.4871, -11.9174) (9.1346, -12.3469) (8.9401, -12.5535) knots 0 0 0 1 2 2 2
  spline S141 degree 2 poles (8.9401, -12.5535) (8.624, -12.8979) (7.8501, -13.6354) (7.6192, -13.8501) knots 0 0 0 1 2 2 2
  line L96 (7.6192, -13.8501) -> (10.0746, -13.8501)
  line L97 (10.0746, -13.8501) -> (10.0746, -14.4295)
  spline S142 degree 2 poles (13.7739, -12.8412) (13.7739, -13.2018) (13.543, -13.8177) (13.3323, -14.0446) knots 0 0 0 1 2 2 2
  spline S143 degree 2 poles (13.3323, -14.0446) (13.1216, -14.2715) (12.4936, -14.5349) (12.1046, -14.5349) knots 0 0 0 1 2 2 2
  spline S144 degree 2 poles (12.1046, -14.5349) (11.748, -14.5349) (11.0511, -14.3769) (10.7958, -14.2513) knots 0 0 0 1 2 2 2
  line L98 (10.7958, -14.2513) -> (10.7958, -13.5422)
  line L99 (10.7958, -13.5422) -> (10.8444, -13.5422)
  spline S145 degree 2 poles (10.8444, -13.5422) (10.9214, -13.5989) (11.2091, -13.7448) (11.3833, -13.8096) knots 0 0 0 1 2 2 2
  spline S146 degree 2 poles (11.3833, -13.8096) (11.5819, -13.8785) (11.9101, -13.9555) (12.1167, -13.9555) knots 0 0 0 1 2 2 2
  spline S147 degree 2 poles (12.1167, -13.9555) (12.3193, -13.9555) (12.7002, -13.8096) (12.838, -13.6516) knots 0 0 0 1 2 2 2
  spline S148 degree 2 poles (12.838, -13.6516) (12.9636, -13.5017) (13.0932, -13.1046) (13.0932, -12.8372) knots 0 0 0 1 2 2 2
  spline S149 degree 2 poles (13.0932, -12.8372) (13.0932, -12.5697) (12.9474, -12.2294) (12.8096, -12.1159) knots 0 0 0 1 2 2 2
  spline S150 degree 2 poles (12.8096, -12.1159) (12.6678, -11.9903) (12.2464, -11.885) (11.9911, -11.885) knots 0 0 0 1 2 2 2
  spline S151 degree 2 poles (11.9911, -11.885) (11.7156, -11.885) (11.1686, -11.9701) (11.0025, -12.0065) knots 0 0 0 1 2 2 2
  line L100 (11.0025, -12.0065) -> (11.0025, -9.4295)
  line L101 (11.0025, -9.4295) -> (13.7456, -9.4295)
  line L102 (13.7456, -9.4295) -> (13.7456, -10.0171)
  line L103 (13.7456, -10.0171) -> (11.6467, -10.0171)
  line L104 (11.6467, -10.0171) -> (11.6467, -11.3501)
  spline S152 degree 2 poles (11.6467, -11.3501) (11.7683, -11.3339) (12.0033, -11.3218) (12.1005, -11.3218) knots 0 0 0 1 2 2 2
  spline S153 degree 2 poles (12.1005, -11.3218) (12.4855, -11.3218) (13.0162, -11.4474) (13.2594, -11.6338) knots 0 0 0 1 2 2 2
  spline S154 degree 2 poles (13.2594, -11.6338) (13.5065, -11.8201) (13.7739, -12.3874) (13.7739, -12.8412) knots 0 0 0 1 2 2 2
  point P0 (0, 0)
  constraints: 2 other
emboss "Emboss1" sketch "Sketch15" operation cut depth 1 direction (0, -1, 0)
equation "\"d87\" = d94"
equation "\"d88\" = 0.160083 * Sketch13_Pitch"
equation "\"d89\" = 0.160083 * Sketch13_Pitch"
equation "\"d92\" = Sketch13_Pitch"
equation "\"d36\" = 55deg"
equation "\"Sketch5_Pitch\" = 1.25"
equation "\"d54\" = 55deg"
equation "\"Sketch7_Pitch\" = 1.25"
equation "\"d74\" = 55deg"
equation "\"Sketch10_Pitch\" = 1.5"
equation "\"d94\" = 55deg"
equation "\"Sketch13_Pitch\" = 1.5"
body "Solid1"
body "Solid5"
